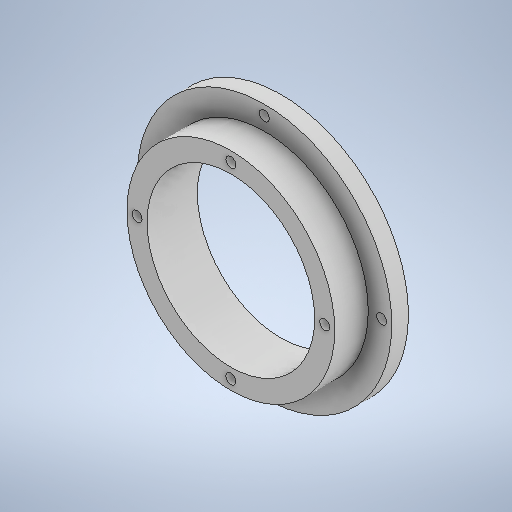
# Autodesk Inventor part: ModuleConnector
Saved by Autodesk Inventor 2025.1 (Build 291241020, 241B)
## iProperties
Created: 2024-09-22
Part Number: ModuleConnector
Material: 일반
Document SubType Name: Modeling
Designer: daare
Density: 1 g/cm^3
Appearance: 기본값
Author: daare
Autodesk Inventor part; units mm, degrees
ref_plane "YZ Plane" through (0, 0, 0) normal (1, 0, 0) x (0, 1, 0)
ref_plane "XZ Plane" through (0, 0, 0) normal (0, 1, 0) x (-1, 0, 0)
ref_plane "XY Plane" through (0, 0, 0) normal (0, 0, 1) x (1, 0, 0)
sketch "스케치1" plane through (0, 0, 0) normal (0, 0, 1) x (1, 0, 0)
  circle A0 centre (0, 0) radius 25
  circle A1 centre (-35, 0) radius 1.5
  circle A2 centre (0, 0) radius 31
  circle A3 centre (0, 0) radius 38
  circle A4 centre (0, -35) radius 1.5
  circle A5 centre (35, 0) radius 1.5
  circle A6 centre (0, 35) radius 1.5
  dimension "d0" = 50
  dimension "d2" = 3
  dimension "d4" = 6
  dimension "d27" = 1.5
  dimension "d28" = 35
  dimension "d31" = 360
  constraints: 7 centre point, 2 coincident, 1 horizontal alignment, 9 other
  measures "d0" diameter of A0
  measures "d2" diameter of A1
  measures "d4" radial gap between concentric circles of A0 A2
  measures "d28" distance of A1.centre point (0, 0)
extrude "돌출1" add sketch "스케치1" along normal blind 5 contours A3
extrude "돌출2" add sketch "스케치1" along normal blind 15 contours A2
sketch "스케치2" plane through (0, 0, 15) normal (0, 0, 1) x (1, 0, 0)
  circle A0 centre (0, 0) radius 25 projected
  circle A1 centre (0, 0) radius 31 projected
  line L0 (-1.611, 31) -> (1.611, 31)
  point P0 (0, 28)
  point P1 (0, 31)
  point P2 (-28, 0)
  point P3 (0, -28)
  point P4 (28, 0)
  dimension "d14" = 6
  dimension "d15" = 3
  dimension "d18" = 360
  constraints: 2 end point, 2 vertical alignment, 1 horizontal, 1 midpoint, 1 tangent, 5 other
  measures "d14" radial gap between concentric circles of A0 A1
  measures "d15" distance from line of point (0, 28) L0
hole "구멍1" at (0, 28, 15) at (-28, 0, 15) at (0, -28, 15) at (28, 0, 15) direction (0, 0, -1) diameter 3 depth 8 tip angle 118
equation "\"d15\" = 0.5 * d14"
